Autodesk Inventor part; units mm, degrees
(part 3 of 6)
  arc A1155 (-87.7296, 1.38) -> (-88.2287, 1.0682) centre (-87.7298, 0.825) ccw
  arc A1156 (-88.2287, 1.0682) -> (-88.3213, 0.7604) centre (-87.3298, 0.63) ccw
  arc A1157 (-88.47, 0.63) -> (-88.3213, 0.7604) centre (-88.47, 0.78) ccw
  line L149 (-88.47, 0.63) -> (-88.9893, 0.63)
  arc A1158 (-89.138, 0.7604) -> (-88.9893, 0.63) centre (-88.9893, 0.78) ccw
  arc A1159 (-89.138, 0.7604) -> (-89.2306, 1.0682) centre (-90.1294, 0.63) ccw
  arc A1160 (-89.2306, 1.0682) -> (-89.7296, 1.38) centre (-89.7294, 0.825) ccw
  arc A1161 (-89.7296, 1.38) -> (-90.2287, 1.0682) centre (-89.7298, 0.825) ccw
  arc A1162 (-90.2287, 1.0682) -> (-90.3213, 0.7604) centre (-89.3298, 0.63) ccw
  arc A1163 (-90.47, 0.63) -> (-90.3213, 0.7604) centre (-90.47, 0.78) ccw
  line L150 (-90.47, 0.63) -> (-90.9893, 0.63)
  arc A1164 (-91.138, 0.7604) -> (-90.9893, 0.63) centre (-90.9893, 0.78) ccw
  arc A1165 (-91.138, 0.7604) -> (-91.2306, 1.0682) centre (-92.1294, 0.63) ccw
  arc A1166 (-91.2306, 1.0682) -> (-91.7296, 1.38) centre (-91.7294, 0.825) ccw
  arc A1167 (-91.7296, 1.38) -> (-92.2287, 1.0682) centre (-91.7298, 0.825) ccw
  arc A1168 (-92.2287, 1.0682) -> (-92.3213, 0.7604) centre (-91.3298, 0.63) ccw
  arc A1169 (-92.47, 0.63) -> (-92.3213, 0.7604) centre (-92.47, 0.78) ccw
  line L151 (-92.47, 0.63) -> (-92.9893, 0.63)
  arc A1170 (-93.138, 0.7604) -> (-92.9893, 0.63) centre (-92.9893, 0.78) ccw
  arc A1171 (-93.138, 0.7604) -> (-93.2306, 1.0682) centre (-94.1294, 0.63) ccw
  arc A1172 (-93.2306, 1.0682) -> (-93.7296, 1.38) centre (-93.7294, 0.825) ccw
  arc A1173 (-93.7296, 1.38) -> (-94.2287, 1.0682) centre (-93.7298, 0.825) ccw
  arc A1174 (-94.2287, 1.0682) -> (-94.3213, 0.7604) centre (-93.3298, 0.63) ccw
  arc A1175 (-94.47, 0.63) -> (-94.3213, 0.7604) centre (-94.47, 0.78) ccw
  line L152 (-94.47, 0.63) -> (-94.9893, 0.63)
  arc A1176 (-95.138, 0.7604) -> (-94.9893, 0.63) centre (-94.9893, 0.78) ccw
  arc A1177 (-95.138, 0.7604) -> (-95.2306, 1.0682) centre (-96.1294, 0.63) ccw
  arc A1178 (-95.2306, 1.0682) -> (-95.7296, 1.38) centre (-95.7294, 0.825) ccw
  arc A1179 (-95.7296, 1.38) -> (-96.2287, 1.0682) centre (-95.7298, 0.825) ccw
  arc A1180 (-96.2287, 1.0682) -> (-96.3213, 0.7604) centre (-95.3298, 0.63) ccw
  arc A1181 (-96.47, 0.63) -> (-96.3213, 0.7604) centre (-96.47, 0.78) ccw
  line L153 (-96.47, 0.63) -> (-96.9893, 0.63)
  arc A1182 (-97.138, 0.7604) -> (-96.9893, 0.63) centre (-96.9893, 0.78) ccw
  arc A1183 (-97.138, 0.7604) -> (-97.2306, 1.0682) centre (-98.1294, 0.63) ccw
  arc A1184 (-97.2306, 1.0682) -> (-97.7296, 1.38) centre (-97.7294, 0.825) ccw
  arc A1185 (-97.7296, 1.38) -> (-98.2287, 1.0682) centre (-97.7298, 0.825) ccw
  arc A1186 (-98.2287, 1.0682) -> (-98.3213, 0.7604) centre (-97.3298, 0.63) ccw
  arc A1187 (-98.47, 0.63) -> (-98.3213, 0.7604) centre (-98.47, 0.78) ccw
  line L154 (-98.47, 0.63) -> (-98.9893, 0.63)
  arc A1188 (-99.138, 0.7604) -> (-98.9893, 0.63) centre (-98.9893, 0.78) ccw
  arc A1189 (-99.138, 0.7604) -> (-99.2306, 1.0682) centre (-100.1294, 0.63) ccw
  arc A1190 (-99.2306, 1.0682) -> (-99.7296, 1.38) centre (-99.7294, 0.825) ccw
  arc A1191 (-99.7296, 1.38) -> (-100.2287, 1.0682) centre (-99.7298, 0.825) ccw
  arc A1192 (-100.2287, 1.0682) -> (-100.3213, 0.7604) centre (-99.3298, 0.63) ccw
  arc A1193 (-100.47, 0.63) -> (-100.3213, 0.7604) centre (-100.47, 0.78) ccw
  line L155 (-100.47, 0.63) -> (-100.9893, 0.63)
  arc A1194 (-101.138, 0.7604) -> (-100.9893, 0.63) centre (-100.9893, 0.78) ccw
  arc A1195 (-101.138, 0.7604) -> (-101.2306, 1.0682) centre (-102.1294, 0.63) ccw
  arc A1196 (-101.2306, 1.0682) -> (-101.7296, 1.38) centre (-101.7294, 0.825) ccw
  arc A1197 (-101.7296, 1.38) -> (-102.2287, 1.0682) centre (-101.7298, 0.825) ccw
  arc A1198 (-102.2287, 1.0682) -> (-102.3213, 0.7604) centre (-101.3298, 0.63) ccw
  arc A1199 (-102.47, 0.63) -> (-102.3213, 0.7604) centre (-102.47, 0.78) ccw
  line L156 (-102.47, 0.63) -> (-102.9893, 0.63)
  arc A1200 (-103.138, 0.7604) -> (-102.9893, 0.63) centre (-102.9893, 0.78) ccw
  arc A1201 (-103.138, 0.7604) -> (-103.2306, 1.0682) centre (-104.1294, 0.63) ccw
  arc A1202 (-103.2306, 1.0682) -> (-103.7296, 1.38) centre (-103.7294, 0.825) ccw
  arc A1203 (-103.7296, 1.38) -> (-104.2287, 1.0682) centre (-103.7298, 0.825) ccw
  arc A1204 (-104.2287, 1.0682) -> (-104.3213, 0.7604) centre (-103.3298, 0.63) ccw
  arc A1205 (-104.47, 0.63) -> (-104.3213, 0.7604) centre (-104.47, 0.78) ccw
  line L157 (-104.47, 0.63) -> (-104.9893, 0.63)
  arc A1206 (-105.138, 0.7604) -> (-104.9893, 0.63) centre (-104.9893, 0.78) ccw
  arc A1207 (-105.138, 0.7604) -> (-105.2306, 1.0682) centre (-106.1294, 0.63) ccw
  arc A1208 (-105.2306, 1.0682) -> (-105.7296, 1.38) centre (-105.7294, 0.825) ccw
  arc A1209 (-105.7296, 1.38) -> (-106.2287, 1.0682) centre (-105.7298, 0.825) ccw
  arc A1210 (-106.2287, 1.0682) -> (-106.3213, 0.7604) centre (-105.3298, 0.63) ccw
  arc A1211 (-106.47, 0.63) -> (-106.3213, 0.7604) centre (-106.47, 0.78) ccw
  line L158 (-106.47, 0.63) -> (-106.9893, 0.63)
  arc A1212 (-107.138, 0.7604) -> (-106.9893, 0.63) centre (-106.9893, 0.78) ccw
  arc A1213 (-107.138, 0.7604) -> (-107.2306, 1.0682) centre (-108.1294, 0.63) ccw
  arc A1214 (-107.2306, 1.0682) -> (-107.7296, 1.38) centre (-107.7294, 0.825) ccw
  arc A1215 (-107.7296, 1.38) -> (-108.2287, 1.0682) centre (-107.7298, 0.825) ccw
  arc A1216 (-108.2287, 1.0682) -> (-108.3213, 0.7604) centre (-107.3298, 0.63) ccw
  arc A1217 (-108.47, 0.63) -> (-108.3213, 0.7604) centre (-108.47, 0.78) ccw
  line L159 (-108.47, 0.63) -> (-108.9893, 0.63)
  arc A1218 (-109.138, 0.7604) -> (-108.9893, 0.63) centre (-108.9893, 0.78) ccw
  arc A1219 (-109.138, 0.7604) -> (-109.2306, 1.0682) centre (-110.1294, 0.63) ccw
  arc A1220 (-109.2306, 1.0682) -> (-109.7296, 1.38) centre (-109.7294, 0.825) ccw
  arc A1221 (-109.7296, 1.38) -> (-110.2287, 1.0682) centre (-109.7298, 0.825) ccw
  arc A1222 (-110.2287, 1.0682) -> (-110.3213, 0.7604) centre (-109.3298, 0.63) ccw
  arc A1223 (-110.47, 0.63) -> (-110.3213, 0.7604) centre (-110.47, 0.78) ccw
  line L160 (-110.47, 0.63) -> (-110.9893, 0.63)
  arc A1224 (-111.138, 0.7604) -> (-110.9893, 0.63) centre (-110.9893, 0.78) ccw
  arc A1225 (-111.138, 0.7604) -> (-111.2306, 1.0682) centre (-112.1294, 0.63) ccw
  arc A1226 (-111.2306, 1.0682) -> (-111.7296, 1.38) centre (-111.7294, 0.825) ccw
  arc A1227 (-111.7296, 1.38) -> (-112.2287, 1.0682) centre (-111.7298, 0.825) ccw
  arc A1228 (-112.2287, 1.0682) -> (-112.3213, 0.7604) centre (-111.3298, 0.63) ccw
  arc A1229 (-112.47, 0.63) -> (-112.3213, 0.7604) centre (-112.47, 0.78) ccw
  line L161 (-112.47, 0.63) -> (-112.9893, 0.63)
  arc A1230 (-113.138, 0.7604) -> (-112.9893, 0.63) centre (-112.9893, 0.78) ccw
  arc A1231 (-113.138, 0.7604) -> (-113.2306, 1.0682) centre (-114.1294, 0.63) ccw
  arc A1232 (-113.2306, 1.0682) -> (-113.7296, 1.38) centre (-113.7294, 0.825) ccw
  arc A1233 (-113.7296, 1.38) -> (-114.2287, 1.0682) centre (-113.7298, 0.825) ccw
  arc A1234 (-114.2287, 1.0682) -> (-114.3213, 0.7604) centre (-113.3298, 0.63) ccw
  arc A1235 (-114.47, 0.63) -> (-114.3213, 0.7604) centre (-114.47, 0.78) ccw
  line L162 (-114.47, 0.63) -> (-114.9893, 0.63)
  arc A1236 (-115.138, 0.7604) -> (-114.9893, 0.63) centre (-114.9893, 0.78) ccw
  arc A1237 (-115.138, 0.7604) -> (-115.2306, 1.0682) centre (-116.1294, 0.63) ccw
  arc A1238 (-115.2306, 1.0682) -> (-115.7296, 1.38) centre (-115.7294, 0.825) ccw
  arc A1239 (-115.7296, 1.38) -> (-116.2287, 1.0682) centre (-115.7298, 0.825) ccw
  arc A1240 (-116.2287, 1.0682) -> (-116.3213, 0.7604) centre (-115.3298, 0.63) ccw
  arc A1241 (-116.47, 0.63) -> (-116.3213, 0.7604) centre (-116.47, 0.78) ccw
  line L163 (-116.47, 0.63) -> (-116.9893, 0.63)
  arc A1242 (-117.138, 0.7604) -> (-116.9893, 0.63) centre (-116.9893, 0.78) ccw
  arc A1243 (-117.138, 0.7604) -> (-117.2306, 1.0682) centre (-118.1294, 0.63) ccw
  arc A1244 (-117.2306, 1.0682) -> (-117.7296, 1.38) centre (-117.7294, 0.825) ccw
  arc A1245 (-117.7296, 1.38) -> (-118.2287, 1.0682) centre (-117.7298, 0.825) ccw
  arc A1246 (-118.2287, 1.0682) -> (-118.3213, 0.7604) centre (-117.3298, 0.63) ccw
  arc A1247 (-118.47, 0.63) -> (-118.3213, 0.7604) centre (-118.47, 0.78) ccw
  line L164 (-118.47, 0.63) -> (-118.9893, 0.63)
  arc A1248 (-119.138, 0.7604) -> (-118.9893, 0.63) centre (-118.9893, 0.78) ccw
  arc A1249 (-119.138, 0.7604) -> (-119.2306, 1.0682) centre (-120.1294, 0.63) ccw
  arc A1250 (-119.2306, 1.0682) -> (-119.7296, 1.38) centre (-119.7294, 0.825) ccw
  arc A1251 (-119.7296, 1.38) -> (-120.2287, 1.0682) centre (-119.7298, 0.825) ccw
  arc A1252 (-120.2287, 1.0682) -> (-120.3213, 0.7604) centre (-119.3298, 0.63) ccw
  arc A1253 (-120.47, 0.63) -> (-120.3213, 0.7604) centre (-120.47, 0.78) ccw
  line L165 (-120.47, 0.63) -> (-120.9893, 0.63)
  arc A1254 (-121.138, 0.7604) -> (-120.9893, 0.63) centre (-120.9893, 0.78) ccw
  arc A1255 (-121.138, 0.7604) -> (-121.2306, 1.0682) centre (-122.1294, 0.63) ccw
  arc A1256 (-121.2306, 1.0682) -> (-121.7296, 1.38) centre (-121.7294, 0.825) ccw
  arc A1257 (-121.7296, 1.38) -> (-122.2287, 1.0682) centre (-121.7298, 0.825) ccw
  arc A1258 (-122.2287, 1.0682) -> (-122.3213, 0.7604) centre (-121.3298, 0.63) ccw
  arc A1259 (-122.47, 0.63) -> (-122.3213, 0.7604) centre (-122.47, 0.78) ccw
  line L166 (-122.47, 0.63) -> (-122.9893, 0.63)
  arc A1260 (-123.138, 0.7604) -> (-122.9893, 0.63) centre (-122.9893, 0.78) ccw
  arc A1261 (-123.138, 0.7604) -> (-123.2306, 1.0682) centre (-124.1294, 0.63) ccw
  arc A1262 (-123.2306, 1.0682) -> (-123.7296, 1.38) centre (-123.7294, 0.825) ccw
  arc A1263 (-123.7296, 1.38) -> (-124.2287, 1.0682) centre (-123.7298, 0.825) ccw
  arc A1264 (-124.2287, 1.0682) -> (-124.3213, 0.7604) centre (-123.3298, 0.63) ccw
  arc A1265 (-124.47, 0.63) -> (-124.3213, 0.7604) centre (-124.47, 0.78) ccw
  line L167 (-124.47, 0.63) -> (-124.9893, 0.63)
  arc A1266 (-125.138, 0.7604) -> (-124.9893, 0.63) centre (-124.9893, 0.78) ccw
  arc A1267 (-125.138, 0.7604) -> (-125.2306, 1.0682) centre (-126.1294, 0.63) ccw
  arc A1268 (-125.2306, 1.0682) -> (-125.7296, 1.38) centre (-125.7294, 0.825) ccw
  arc A1269 (-125.7296, 1.38) -> (-126.2287, 1.0682) centre (-125.7298, 0.825) ccw
  arc A1270 (-126.2287, 1.0682) -> (-126.3213, 0.7604) centre (-125.3298, 0.63) ccw
  arc A1271 (-126.47, 0.63) -> (-126.3213, 0.7604) centre (-126.47, 0.78) ccw
  line L168 (-126.47, 0.63) -> (-126.9893, 0.63)
  arc A1272 (-127.138, 0.7604) -> (-126.9893, 0.63) centre (-126.9893, 0.78) ccw
  arc A1273 (-127.138, 0.7604) -> (-127.2306, 1.0682) centre (-128.1294, 0.63) ccw
  arc A1274 (-127.2306, 1.0682) -> (-127.7296, 1.38) centre (-127.7294, 0.825) ccw
  arc A1275 (-127.7296, 1.38) -> (-128.2287, 1.0682) centre (-127.7298, 0.825) ccw
  arc A1276 (-128.2287, 1.0682) -> (-128.3213, 0.7604) centre (-127.3298, 0.63) ccw
  arc A1277 (-128.47, 0.63) -> (-128.3213, 0.7604) centre (-128.47, 0.78) ccw
  line L169 (-128.47, 0.63) -> (-128.9893, 0.63)
  arc A1278 (-129.138, 0.7604) -> (-128.9893, 0.63) centre (-128.9893, 0.78) ccw
  arc A1279 (-129.138, 0.7604) -> (-129.2306, 1.0682) centre (-130.1294, 0.63) ccw
  arc A1280 (-129.2306, 1.0682) -> (-129.7296, 1.38) centre (-129.7294, 0.825) ccw
  arc A1281 (-129.7296, 1.38) -> (-130.2287, 1.0682) centre (-129.7298, 0.825) ccw
  arc A1282 (-130.2287, 1.0682) -> (-130.3213, 0.7604) centre (-129.3298, 0.63) ccw
  arc A1283 (-130.47, 0.63) -> (-130.3213, 0.7604) centre (-130.47, 0.78) ccw
  line L170 (-130.47, 0.63) -> (-130.9893, 0.63)
  arc A1284 (-131.138, 0.7604) -> (-130.9893, 0.63) centre (-130.9893, 0.78) ccw
  arc A1285 (-131.138, 0.7604) -> (-131.2306, 1.0682) centre (-132.1294, 0.63) ccw
  arc A1286 (-131.2306, 1.0682) -> (-131.7296, 1.38) centre (-131.7294, 0.825) ccw
  arc A1287 (-131.7296, 1.38) -> (-132.2287, 1.0682) centre (-131.7298, 0.825) ccw
  arc A1288 (-132.2287, 1.0682) -> (-132.3213, 0.7604) centre (-131.3298, 0.63) ccw
  arc A1289 (-132.47, 0.63) -> (-132.3213, 0.7604) centre (-132.47, 0.78) ccw
  line L171 (-132.47, 0.63) -> (-132.9893, 0.63)
  arc A1290 (-133.138, 0.7604) -> (-132.9893, 0.63) centre (-132.9893, 0.78) ccw
  arc A1291 (-133.138, 0.7604) -> (-133.2306, 1.0682) centre (-134.1294, 0.63) ccw
  arc A1292 (-133.2306, 1.0682) -> (-133.7296, 1.38) centre (-133.7294, 0.825) ccw
  arc A1293 (-133.7296, 1.38) -> (-134.2287, 1.0682) centre (-133.7298, 0.825) ccw
  arc A1294 (-134.2287, 1.0682) -> (-134.3213, 0.7604) centre (-133.3298, 0.63) ccw
  arc A1295 (-134.47, 0.63) -> (-134.3213, 0.7604) centre (-134.47, 0.78) ccw
  line L172 (-134.47, 0.63) -> (-134.9893, 0.63)
  arc A1296 (-135.138, 0.7604) -> (-134.9893, 0.63) centre (-134.9893, 0.78) ccw
  arc A1297 (-135.138, 0.7604) -> (-135.2306, 1.0682) centre (-136.1294, 0.63) ccw
  arc A1298 (-135.2306, 1.0682) -> (-135.7296, 1.38) centre (-135.7294, 0.825) ccw
  arc A1299 (-135.7296, 1.38) -> (-136.2287, 1.0682) centre (-135.7298, 0.825) ccw
  arc A1300 (-136.2287, 1.0682) -> (-136.3213, 0.7604) centre (-135.3298, 0.63) ccw
  arc A1301 (-136.47, 0.63) -> (-136.3213, 0.7604) centre (-136.47, 0.78) ccw
  line L173 (-136.47, 0.63) -> (-136.9893, 0.63)
  arc A1302 (-137.138, 0.7604) -> (-136.9893, 0.63) centre (-136.9893, 0.78) ccw
  arc A1303 (-137.138, 0.7604) -> (-137.2306, 1.0682) centre (-138.1294, 0.63) ccw
  arc A1304 (-137.2306, 1.0682) -> (-137.7296, 1.38) centre (-137.7294, 0.825) ccw
  arc A1305 (-137.7296, 1.38) -> (-138.2287, 1.0682) centre (-137.7298, 0.825) ccw
  arc A1306 (-138.2287, 1.0682) -> (-138.3213, 0.7604) centre (-137.3298, 0.63) ccw
  arc A1307 (-138.47, 0.63) -> (-138.3213, 0.7604) centre (-138.47, 0.78) ccw
  line L174 (-138.47, 0.63) -> (-138.9893, 0.63)
  arc A1308 (-139.138, 0.7604) -> (-138.9893, 0.63) centre (-138.9893, 0.78) ccw
  arc A1309 (-139.138, 0.7604) -> (-139.2306, 1.0682) centre (-140.1294, 0.63) ccw
  arc A1310 (-139.2306, 1.0682) -> (-139.7296, 1.38) centre (-139.7294, 0.825) ccw
  arc A1311 (-139.7296, 1.38) -> (-140.2287, 1.0682) centre (-139.7298, 0.825) ccw
  arc A1312 (-140.2287, 1.0682) -> (-140.3213, 0.7604) centre (-139.3298, 0.63) ccw
  arc A1313 (-140.47, 0.63) -> (-140.3213, 0.7604) centre (-140.47, 0.78) ccw
  line L175 (-140.47, 0.63) -> (-140.9893, 0.63)
  arc A1314 (-141.138, 0.7604) -> (-140.9893, 0.63) centre (-140.9893, 0.78) ccw
  arc A1315 (-141.138, 0.7604) -> (-141.2306, 1.0682) centre (-142.1294, 0.63) ccw
  arc A1316 (-141.2306, 1.0682) -> (-141.7296, 1.38) centre (-141.7294, 0.825) ccw
  arc A1317 (-141.7296, 1.38) -> (-142.2287, 1.0682) centre (-141.7298, 0.825) ccw
  arc A1318 (-142.2287, 1.0682) -> (-142.3213, 0.7604) centre (-141.3298, 0.63) ccw
  arc A1319 (-142.47, 0.63) -> (-142.3213, 0.7604) centre (-142.47, 0.78) ccw
  line L176 (-142.47, 0.63) -> (-142.9893, 0.63)
  arc A1320 (-143.138, 0.7604) -> (-142.9893, 0.63) centre (-142.9893, 0.78) ccw
  arc A1321 (-143.138, 0.7604) -> (-143.2306, 1.0682) centre (-144.1294, 0.63) ccw
  arc A1322 (-143.2306, 1.0682) -> (-143.7296, 1.38) centre (-143.7294, 0.825) ccw
  arc A1323 (-143.7296, 1.38) -> (-144.2287, 1.0682) centre (-143.7298, 0.825) ccw
  arc A1324 (-144.2287, 1.0682) -> (-144.3213, 0.7604) centre (-143.3298, 0.63) ccw
  arc A1325 (-144.47, 0.63) -> (-144.3213, 0.7604) centre (-144.47, 0.78) ccw
  line L177 (-144.47, 0.63) -> (-144.9893, 0.63)
  arc A1326 (-145.138, 0.7604) -> (-144.9893, 0.63) centre (-144.9893, 0.78) ccw
  arc A1327 (-145.138, 0.7604) -> (-145.2306, 1.0682) centre (-146.1294, 0.63) ccw
  arc A1328 (-145.2306, 1.0682) -> (-145.7296, 1.38) centre (-145.7294, 0.825) ccw
  arc A1329 (-145.7296, 1.38) -> (-146.2287, 1.0682) centre (-145.7298, 0.825) ccw
  arc A1330 (-146.2287, 1.0682) -> (-146.3213, 0.7604) centre (-145.3298, 0.63) ccw
  arc A1331 (-146.47, 0.63) -> (-146.3213, 0.7604) centre (-146.47, 0.78) ccw
  line L178 (-146.47, 0.63) -> (-146.9893, 0.63)
  arc A1332 (-147.138, 0.7604) -> (-146.9893, 0.63) centre (-146.9893, 0.78) ccw
  arc A1333 (-147.138, 0.7604) -> (-147.2306, 1.0682) centre (-148.1294, 0.63) ccw
  arc A1334 (-147.2306, 1.0682) -> (-147.7296, 1.38) centre (-147.7294, 0.825) ccw
  arc A1335 (-147.7296, 1.38) -> (-148.2287, 1.0682) centre (-147.7298, 0.825) ccw
  arc A1336 (-148.2287, 1.0682) -> (-148.3213, 0.7604) centre (-147.3298, 0.63) ccw
  arc A1337 (-148.47, 0.63) -> (-148.3213, 0.7604) centre (-148.47, 0.78) ccw
  line L179 (-148.47, 0.63) -> (-148.9893, 0.63)
  arc A1338 (-149.138, 0.7604) -> (-148.9893, 0.63) centre (-148.9893, 0.78) ccw
  arc A1339 (-149.138, 0.7604) -> (-149.2306, 1.0682) centre (-150.1294, 0.63) ccw
  arc A1340 (-149.2306, 1.0682) -> (-149.7296, 1.38) centre (-149.7294, 0.825) ccw
  arc A1341 (-149.7296, 1.38) -> (-150.2287, 1.0682) centre (-149.7298, 0.825) ccw
  arc A1342 (-150.2287, 1.0682) -> (-150.3213, 0.7604) centre (-149.3298, 0.63) ccw
  arc A1343 (-150.47, 0.63) -> (-150.3213, 0.7604) centre (-150.47, 0.78) ccw
  line L180 (-150.47, 0.63) -> (-150.9893, 0.63)
  arc A1344 (-151.138, 0.7604) -> (-150.9893, 0.63) centre (-150.9893, 0.78) ccw
  arc A1345 (-151.138, 0.7604) -> (-151.2306, 1.0682) centre (-152.1294, 0.63) ccw
  arc A1346 (-151.2306, 1.0682) -> (-151.7296, 1.38) centre (-151.7294, 0.825) ccw
  arc A1347 (-151.7296, 1.38) -> (-152.2287, 1.0682) centre (-151.7298, 0.825) ccw
  arc A1348 (-152.2287, 1.0682) -> (-152.3213, 0.7604) centre (-151.3298, 0.63) ccw
  arc A1349 (-152.47, 0.63) -> (-152.3213, 0.7604) centre (-152.47, 0.78) ccw
  line L181 (-152.47, 0.63) -> (-152.9893, 0.63)
  arc A1350 (-153.138, 0.7604) -> (-152.9893, 0.63) centre (-152.9893, 0.78) ccw
  arc A1351 (-153.138, 0.7604) -> (-153.2306, 1.0682) centre (-154.1294, 0.63) ccw
  arc A1352 (-153.2306, 1.0682) -> (-153.7296, 1.38) centre (-153.7294, 0.825) ccw
  arc A1353 (-153.7296, 1.38) -> (-154.2287, 1.0682) centre (-153.7298, 0.825) ccw
  arc A1354 (-154.2287, 1.0682) -> (-154.3213, 0.7604) centre (-153.3298, 0.63) ccw
  arc A1355 (-154.47, 0.63) -> (-154.3213, 0.7604) centre (-154.47, 0.78) ccw
  line L182 (-154.47, 0.63) -> (-154.9893, 0.63)
  arc A1356 (-155.138, 0.7604) -> (-154.9893, 0.63) centre (-154.9893, 0.78) ccw
  arc A1357 (-155.138, 0.7604) -> (-155.2306, 1.0682) centre (-156.1294, 0.63) ccw
  arc A1358 (-155.2306, 1.0682) -> (-155.7296, 1.38) centre (-155.7294, 0.825) ccw
  arc A1359 (-155.7296, 1.38) -> (-156.2287, 1.0682) centre (-155.7298, 0.825) ccw
  arc A1360 (-156.2287, 1.0682) -> (-156.3213, 0.7604) centre (-155.3298, 0.63) ccw
  arc A1361 (-156.47, 0.63) -> (-156.3213, 0.7604) centre (-156.47, 0.78) ccw
  line L183 (-156.47, 0.63) -> (-156.9893, 0.63)
  arc A1362 (-157.138, 0.7604) -> (-156.9893, 0.63) centre (-156.9893, 0.78) ccw
  arc A1363 (-157.138, 0.7604) -> (-157.2306, 1.0682) centre (-158.1294, 0.63) ccw
  arc A1364 (-157.2306, 1.0682) -> (-157.7296, 1.38) centre (-157.7294, 0.825) ccw
  arc A1365 (-157.7296, 1.38) -> (-158.2287, 1.0682) centre (-157.7298, 0.825) ccw
  arc A1366 (-158.2287, 1.0682) -> (-158.3213, 0.7604) centre (-157.3298, 0.63) ccw
  arc A1367 (-158.47, 0.63) -> (-158.3213, 0.7604) centre (-158.47, 0.78) ccw
  line L184 (-158.47, 0.63) -> (-158.9893, 0.63)
  arc A1368 (-159.138, 0.7604) -> (-158.9893, 0.63) centre (-158.9893, 0.78) ccw
  arc A1369 (-159.138, 0.7604) -> (-159.2306, 1.0682) centre (-160.1294, 0.63) ccw
  arc A1370 (-159.2306, 1.0682) -> (-159.7296, 1.38) centre (-159.7294, 0.825) ccw
  arc A1371 (-159.7296, 1.38) -> (-160.2287, 1.0682) centre (-159.7298, 0.825) ccw
  arc A1372 (-160.2287, 1.0682) -> (-160.3213, 0.7604) centre (-159.3298, 0.63) ccw
  arc A1373 (-160.47, 0.63) -> (-160.3213, 0.7604) centre (-160.47, 0.78) ccw
  line L185 (-160.47, 0.63) -> (-160.9893, 0.63)
  arc A1374 (-161.138, 0.7604) -> (-160.9893, 0.63) centre (-160.9893, 0.78) ccw
  arc A1375 (-161.138, 0.7604) -> (-161.2306, 1.0682) centre (-162.1294, 0.63) ccw
  arc A1376 (-161.2306, 1.0682) -> (-161.7296, 1.38) centre (-161.7294, 0.825) ccw
  arc A1377 (-161.7296, 1.38) -> (-162.2287, 1.0682) centre (-161.7298, 0.825) ccw
  arc A1378 (-162.2287, 1.0682) -> (-162.3213, 0.7604) centre (-161.3298, 0.63) ccw
  arc A1379 (-162.47, 0.63) -> (-162.3213, 0.7604) centre (-162.47, 0.78) ccw
  line L186 (-162.47, 0.63) -> (-162.9893, 0.63)
  arc A1380 (-163.138, 0.7604) -> (-162.9893, 0.63) centre (-162.9893, 0.78) ccw
  arc A1381 (-163.138, 0.7604) -> (-163.2306, 1.0682) centre (-164.1294, 0.63) ccw
  arc A1382 (-163.2306, 1.0682) -> (-163.7296, 1.38) centre (-163.7294, 0.825) ccw
  arc A1383 (-163.7296, 1.38) -> (-164.2287, 1.0682) centre (-163.7298, 0.825) ccw
  arc A1384 (-164.2287, 1.0682) -> (-164.3213, 0.7604) centre (-163.3298, 0.63) ccw
  arc A1385 (-164.47, 0.63) -> (-164.3213, 0.7604) centre (-164.47, 0.78) ccw
  line L187 (-164.47, 0.63) -> (-164.9893, 0.63)
  arc A1386 (-165.138, 0.7604) -> (-164.9893, 0.63) centre (-164.9893, 0.78) ccw
  arc A1387 (-165.138, 0.7604) -> (-165.2306, 1.0682) centre (-166.1294, 0.63) ccw
  arc A1388 (-165.2306, 1.0682) -> (-165.7296, 1.38) centre (-165.7294, 0.825) ccw
  arc A1389 (-165.7296, 1.38) -> (-166.2287, 1.0682) centre (-165.7298, 0.825) ccw
  arc A1390 (-166.2287, 1.0682) -> (-166.3213, 0.7604) centre (-165.3298, 0.63) ccw
  arc A1391 (-166.47, 0.63) -> (-166.3213, 0.7604) centre (-166.47, 0.78) ccw
  line L188 (-166.47, 0.63) -> (-166.9893, 0.63)
  arc A1392 (-167.138, 0.7604) -> (-166.9893, 0.63) centre (-166.9893, 0.78) ccw
  arc A1393 (-167.138, 0.7604) -> (-167.2306, 1.0682) centre (-168.1294, 0.63) ccw
  arc A1394 (-167.2306, 1.0682) -> (-167.7296, 1.38) centre (-167.7294, 0.825) ccw
  arc A1395 (-167.7296, 1.38) -> (-168.2287, 1.0682) centre (-167.7298, 0.825) ccw
  arc A1396 (-168.2287, 1.0682) -> (-168.3213, 0.7604) centre (-167.3298, 0.63) ccw
  arc A1397 (-168.47, 0.63) -> (-168.3213, 0.7604) centre (-168.47, 0.78) ccw
  line L189 (-168.47, 0.63) -> (-168.9893, 0.63)
  arc A1398 (-169.138, 0.7604) -> (-168.9893, 0.63) centre (-168.9893, 0.78) ccw
  arc A1399 (-169.138, 0.7604) -> (-169.2306, 1.0682) centre (-170.1294, 0.63) ccw
  arc A1400 (-169.2306, 1.0682) -> (-169.7296, 1.38) centre (-169.7294, 0.825) ccw
  arc A1401 (-169.7296, 1.38) -> (-170.2287, 1.0682) centre (-169.7298, 0.825) ccw
  arc A1402 (-170.2287, 1.0682) -> (-170.3213, 0.7604) centre (-169.3298, 0.63) ccw
  arc A1403 (-170.47, 0.63) -> (-170.3213, 0.7604) centre (-170.47, 0.78) ccw
  line L190 (-170.47, 0.63) -> (-170.9893, 0.63)
  arc A1404 (-171.138, 0.7604) -> (-170.9893, 0.63) centre (-170.9893, 0.78) ccw
  arc A1405 (-171.138, 0.7604) -> (-171.2306, 1.0682) centre (-172.1294, 0.63) ccw
  arc A1406 (-171.2306, 1.0682) -> (-171.7296, 1.38) centre (-171.7294, 0.825) ccw
  arc A1407 (-171.7296, 1.38) -> (-172.2287, 1.0682) centre (-171.7298, 0.825) ccw
  arc A1408 (-172.2287, 1.0682) -> (-172.3213, 0.7604) centre (-171.3298, 0.63) ccw
  arc A1409 (-172.47, 0.63) -> (-172.3213, 0.7604) centre (-172.47, 0.78) ccw
  line L191 (-172.47, 0.63) -> (-172.9893, 0.63)
  arc A1410 (-173.138, 0.7604) -> (-172.9893, 0.63) centre (-172.9893, 0.78) ccw
  arc A1411 (-173.138, 0.7604) -> (-173.2306, 1.0682) centre (-174.1294, 0.63) ccw
  arc A1412 (-173.2306, 1.0682) -> (-173.7296, 1.38) centre (-173.7294, 0.825) ccw
  arc A1413 (-173.7296, 1.38) -> (-174.2287, 1.0682) centre (-173.7298, 0.825) ccw
  arc A1414 (-174.2287, 1.0682) -> (-174.3213, 0.7604) centre (-173.3298, 0.63) ccw
  arc A1415 (-174.47, 0.63) -> (-174.3213, 0.7604) centre (-174.47, 0.78) ccw
  line L192 (-174.47, 0.63) -> (-174.9893, 0.63)
  arc A1416 (-175.138, 0.7604) -> (-174.9893, 0.63) centre (-174.9893, 0.78) ccw
  arc A1417 (-175.138, 0.7604) -> (-175.2306, 1.0682) centre (-176.1294, 0.63) ccw
  arc A1418 (-175.2306, 1.0682) -> (-175.7296, 1.38) centre (-175.7294, 0.825) ccw
  arc A1419 (-175.7296, 1.38) -> (-176.2287, 1.0682) centre (-175.7298, 0.825) ccw
  arc A1420 (-176.2287, 1.0682) -> (-176.3213, 0.7604) centre (-175.3298, 0.63) ccw
  arc A1421 (-176.47, 0.63) -> (-176.3213, 0.7604) centre (-176.47, 0.78) ccw
  line L193 (-176.47, 0.63) -> (-176.9893, 0.63)
  arc A1422 (-177.138, 0.7604) -> (-176.9893, 0.63) centre (-176.9893, 0.78) ccw
  arc A1423 (-177.138, 0.7604) -> (-177.2306, 1.0682) centre (-178.1294, 0.63) ccw
  arc A1424 (-177.2306, 1.0682) -> (-177.7296, 1.38) centre (-177.7294, 0.825) ccw
  arc A1425 (-177.7296, 1.38) -> (-178.2287, 1.0682) centre (-177.7298, 0.825) ccw
  arc A1426 (-178.2287, 1.0682) -> (-178.3213, 0.7604) centre (-177.3298, 0.63) ccw
  arc A1427 (-178.47, 0.63) -> (-178.3213, 0.7604) centre (-178.47, 0.78) ccw
  line L194 (-178.47, 0.63) -> (-178.9893, 0.63)
  arc A1428 (-179.138, 0.7604) -> (-178.9893, 0.63) centre (-178.9893, 0.78) ccw
  arc A1429 (-179.138, 0.7604) -> (-179.2306, 1.0682) centre (-180.1294, 0.63) ccw
  arc A1430 (-179.2306, 1.0682) -> (-179.7296, 1.38) centre (-179.7294, 0.825) ccw
  arc A1431 (-179.7296, 1.38) -> (-180.2287, 1.0682) centre (-179.7298, 0.825) ccw
  arc A1432 (-180.2287, 1.0682) -> (-180.3213, 0.7604) centre (-179.3298, 0.63) ccw
  arc A1433 (-180.47, 0.63) -> (-180.3213, 0.7604) centre (-180.47, 0.78) ccw
  line L195 (-180.47, 0.63) -> (-180.9893, 0.63)
  arc A1434 (-181.138, 0.7604) -> (-180.9893, 0.63) centre (-180.9893, 0.78) ccw
  arc A1435 (-181.138, 0.7604) -> (-181.2306, 1.0682) centre (-182.1294, 0.63) ccw
  arc A1436 (-181.2306, 1.0682) -> (-181.7296, 1.38) centre (-181.7294, 0.825) ccw
  arc A1437 (-181.7296, 1.38) -> (-182.2287, 1.0682) centre (-181.7298, 0.825) ccw
  arc A1438 (-182.2287, 1.0682) -> (-182.3213, 0.7604) centre (-181.3298, 0.63) ccw
  arc A1439 (-182.47, 0.63) -> (-182.3213, 0.7604) centre (-182.47, 0.78) ccw
  line L196 (-182.47, 0.63) -> (-182.9893, 0.63)
  arc A1440 (-183.138, 0.7604) -> (-182.9893, 0.63) centre (-182.9893, 0.78) ccw
  arc A1441 (-183.138, 0.7604) -> (-183.2306, 1.0682) centre (-184.1294, 0.63) ccw
  arc A1442 (-183.2306, 1.0682) -> (-183.7296, 1.38) centre (-183.7294, 0.825) ccw
  arc A1443 (-183.7296, 1.38) -> (-184.2287, 1.0682) centre (-183.7298, 0.825) ccw
  arc A1444 (-184.2287, 1.0682) -> (-184.3213, 0.7604) centre (-183.3298, 0.63) ccw
  arc A1445 (-184.47, 0.63) -> (-184.3213, 0.7604) centre (-184.47, 0.78) ccw
  line L197 (-184.47, 0.63) -> (-184.9893, 0.63)
  arc A1446 (-185.138, 0.7604) -> (-184.9893, 0.63) centre (-184.9893, 0.78) ccw
  arc A1447 (-185.138, 0.7604) -> (-185.2306, 1.0682) centre (-186.1294, 0.63) ccw
  arc A1448 (-185.2306, 1.0682) -> (-185.7296, 1.38) centre (-185.7294, 0.825) ccw
  arc A1449 (-185.7296, 1.38) -> (-186.2287, 1.0682) centre (-185.7298, 0.825) ccw
  arc A1450 (-186.2287, 1.0682) -> (-186.3213, 0.7604) centre (-185.3298, 0.63) ccw
  arc A1451 (-186.47, 0.63) -> (-186.3213, 0.7604) centre (-186.47, 0.78) ccw
  line L198 (-186.47, 0.63) -> (-186.9893, 0.63)
  arc A1452 (-187.138, 0.7604) -> (-186.9893, 0.63) centre (-186.9893, 0.78) ccw
  arc A1453 (-187.138, 0.7604) -> (-187.2306, 1.0682) centre (-188.1294, 0.63) ccw
  arc A1454 (-187.2306, 1.0682) -> (-187.7296, 1.38) centre (-187.7294, 0.825) ccw
  arc A1455 (-187.7296, 1.38) -> (-188.2287, 1.0682) centre (-187.7298, 0.825) ccw
  arc A1456 (-188.2287, 1.0682) -> (-188.3213, 0.7604) centre (-187.3298, 0.63) ccw
  arc A1457 (-188.47, 0.63) -> (-188.3213, 0.7604) centre (-188.47, 0.78) ccw
  line L199 (-188.47, 0.63) -> (-188.9893, 0.63)
  arc A1458 (-189.138, 0.7604) -> (-188.9893, 0.63) centre (-188.9893, 0.78) ccw
  arc A1459 (-189.138, 0.7604) -> (-189.2306, 1.0682) centre (-190.1294, 0.63) ccw
  arc A1460 (-189.2306, 1.0682) -> (-189.7296, 1.38) centre (-189.7294, 0.825) ccw
  arc A1461 (-189.7296, 1.38) -> (-190.2287, 1.0682) centre (-189.7298, 0.825) ccw
  arc A1462 (-190.2287, 1.0682) -> (-190.3213, 0.7604) centre (-189.3298, 0.63) ccw
  arc A1463 (-190.47, 0.63) -> (-190.3213, 0.7604) centre (-190.47, 0.78) ccw
  line L200 (-190.47, 0.63) -> (-190.9893, 0.63)
  arc A1464 (-191.138, 0.7604) -> (-190.9893, 0.63) centre (-190.9893, 0.78) ccw
  arc A1465 (-191.138, 0.7604) -> (-191.2306, 1.0682) centre (-192.1294, 0.63) ccw
  arc A1466 (-191.2306, 1.0682) -> (-191.7296, 1.38) centre (-191.7294, 0.825) ccw
  arc A1467 (-191.7296, 1.38) -> (-192.2287, 1.0682) centre (-191.7298, 0.825) ccw
  arc A1468 (-192.2287, 1.0682) -> (-192.3213, 0.7604) centre (-191.3298, 0.63) ccw
  arc A1469 (-192.47, 0.63) -> (-192.3213, 0.7604) centre (-192.47, 0.78) ccw
  line L201 (-192.47, 0.63) -> (-192.9893, 0.63)
  arc A1470 (-193.138, 0.7604) -> (-192.9893, 0.63) centre (-192.9893, 0.78) ccw
  arc A1471 (-193.138, 0.7604) -> (-193.2306, 1.0682) centre (-194.1294, 0.63) ccw
  arc A1472 (-193.2306, 1.0682) -> (-193.7296, 1.38) centre (-193.7294, 0.825) ccw
  arc A1473 (-193.7296, 1.38) -> (-194.2287, 1.0682) centre (-193.7298, 0.825) ccw
  arc A1474 (-194.2287, 1.0682) -> (-194.3213, 0.7604) centre (-193.3298, 0.63) ccw
  arc A1475 (-194.47, 0.63) -> (-194.3213, 0.7604) centre (-194.47, 0.78) ccw
  line L202 (-194.47, 0.63) -> (-194.9893, 0.63)
  arc A1476 (-195.138, 0.7604) -> (-194.9893, 0.63) centre (-194.9893, 0.78) ccw
  arc A1477 (-195.138, 0.7604) -> (-195.2306, 1.0682) centre (-196.1294, 0.63) ccw
  arc A1478 (-195.2306, 1.0682) -> (-195.7296, 1.38) centre (-195.7294, 0.825) ccw
  arc A1479 (-195.7296, 1.38) -> (-196.2287, 1.0682) centre (-195.7298, 0.825) ccw
  arc A1480 (-196.2287, 1.0682) -> (-196.3213, 0.7604) centre (-195.3298, 0.63) ccw
  arc A1481 (-196.47, 0.63) -> (-196.3213, 0.7604) centre (-196.47, 0.78) ccw
  line L203 (-196.47, 0.63) -> (-196.9893, 0.63)
  arc A1482 (-197.138, 0.7604) -> (-196.9893, 0.63) centre (-196.9893, 0.78) ccw
  arc A1483 (-197.138, 0.7604) -> (-197.2306, 1.0682) centre (-198.1294, 0.63) ccw
  arc A1484 (-197.2306, 1.0682) -> (-197.7296, 1.38) centre (-197.7294, 0.825) ccw
  arc A1485 (-197.7296, 1.38) -> (-198.2287, 1.0682) centre (-197.7298, 0.825) ccw
  arc A1486 (-198.2287, 1.0682) -> (-198.3213, 0.7604) centre (-197.3298, 0.63) ccw
  arc A1487 (-198.47, 0.63) -> (-198.3213, 0.7604) centre (-198.47, 0.78) ccw
  line L204 (-198.47, 0.63) -> (-198.9893, 0.63)
  arc A1488 (-199.138, 0.7604) -> (-198.9893, 0.63) centre (-198.9893, 0.78) ccw
  arc A1489 (-199.138, 0.7604) -> (-199.2306, 1.0682) centre (-200.1294, 0.63) ccw
  arc A1490 (-199.2306, 1.0682) -> (-199.7296, 1.38) centre (-199.7294, 0.825) ccw
  arc A1491 (-199.7296, 1.38) -> (-200.2287, 1.0682) centre (-199.7298, 0.825) ccw
  arc A1492 (-200.2287, 1.0682) -> (-200.3213, 0.7604) centre (-199.3298, 0.63) ccw
  arc A1493 (-200.47, 0.63) -> (-200.3213, 0.7604) centre (-200.47, 0.78) ccw
  line L205 (-200.47, 0.63) -> (-200.9893, 0.63)
  arc A1494 (-201.138, 0.7604) -> (-200.9893, 0.63) centre (-200.9893, 0.78) ccw
  arc A1495 (-201.138, 0.7604) -> (-201.2306, 1.0682) centre (-202.1294, 0.63) ccw
  arc A1496 (-201.2306, 1.0682) -> (-201.7296, 1.38) centre (-201.7294, 0.825) ccw
  arc A1497 (-201.7296, 1.38) -> (-202.2287, 1.0682) centre (-201.7298, 0.825) ccw
  arc A1498 (-202.2287, 1.0682) -> (-202.3213, 0.7604) centre (-201.3298, 0.63) ccw
  arc A1499 (-202.47, 0.63) -> (-202.3213, 0.7604) centre (-202.47, 0.78) ccw
  line L206 (-202.47, 0.63) -> (-202.9893, 0.63)
  arc A1500 (-203.138, 0.7604) -> (-202.9893, 0.63) centre (-202.9893, 0.78) ccw
  arc A1501 (-203.138, 0.7604) -> (-203.2306, 1.0682) centre (-204.1294, 0.63) ccw
  arc A1502 (-203.2306, 1.0682) -> (-203.7296, 1.38) centre (-203.7294, 0.825) ccw
  arc A1503 (-203.7296, 1.38) -> (-204.2287, 1.0682) centre (-203.7298, 0.825) ccw
  arc A1504 (-204.2287, 1.0682) -> (-204.3213, 0.7604) centre (-203.3298, 0.63) ccw
  arc A1505 (-204.47, 0.63) -> (-204.3213, 0.7604) centre (-204.47, 0.78) ccw
  line L207 (-204.47, 0.63) -> (-204.9893, 0.63)
  arc A1506 (-205.138, 0.7604) -> (-204.9893, 0.63) centre (-204.9893, 0.78) ccw
  arc A1507 (-205.138, 0.7604) -> (-205.2306, 1.0682) centre (-206.1294, 0.63) ccw
  arc A1508 (-205.2306, 1.0682) -> (-205.7296, 1.38) centre (-205.7294, 0.825) ccw
  arc A1509 (-205.7296, 1.38) -> (-206.2287, 1.0682) centre (-205.7298, 0.825) ccw
  arc A1510 (-206.2287, 1.0682) -> (-206.3213, 0.7604) centre (-205.3298, 0.63) ccw
  arc A1511 (-206.47, 0.63) -> (-206.3213, 0.7604) centre (-206.47, 0.78) ccw
  line L208 (-206.47, 0.63) -> (-206.9893, 0.63)
  arc A1512 (-207.138, 0.7604) -> (-206.9893, 0.63) centre (-206.9893, 0.78) ccw
  arc A1513 (-207.138, 0.7604) -> (-207.2306, 1.0682) centre (-208.1294, 0.63) ccw
  arc A1514 (-207.2306, 1.0682) -> (-207.7296, 1.38) centre (-207.7294, 0.825) ccw
  arc A1515 (-207.7296, 1.38) -> (-208.2287, 1.0682) centre (-207.7298, 0.825) ccw
  arc A1516 (-208.2287, 1.0682) -> (-208.3213, 0.7604) centre (-207.3298, 0.63) ccw
  arc A1517 (-208.47, 0.63) -> (-208.3213, 0.7604) centre (-208.47, 0.78) ccw
  line L209 (-208.47, 0.63) -> (-208.9893, 0.63)
  arc A1518 (-209.138, 0.7604) -> (-208.9893, 0.63) centre (-208.9893, 0.78) ccw
  arc A1519 (-209.138, 0.7604) -> (-209.2306, 1.0682) centre (-210.1294, 0.63) ccw
  arc A1520 (-209.2306, 1.0682) -> (-209.7296, 1.38) centre (-209.7294, 0.825) ccw
  arc A1521 (-209.7296, 1.38) -> (-210.2287, 1.0682) centre (-209.7298, 0.825) ccw
  arc A1522 (-210.2287, 1.0682) -> (-210.3213, 0.7604) centre (-209.3298, 0.63) ccw
  arc A1523 (-210.47, 0.63) -> (-210.3213, 0.7604) centre (-210.47, 0.78) ccw
  line L210 (-210.47, 0.63) -> (-210.9893, 0.63)
  arc A1524 (-211.138, 0.7604) -> (-210.9893, 0.63) centre (-210.9893, 0.78) ccw
  arc A1525 (-211.138, 0.7604) -> (-211.2306, 1.0682) centre (-212.1294, 0.63) ccw
  arc A1526 (-211.2306, 1.0682) -> (-211.7296, 1.38) centre (-211.7294, 0.825) ccw
  arc A1527 (-211.7296, 1.38) -> (-212.2287, 1.0682) centre (-211.7298, 0.825) ccw
  arc A1528 (-212.2287, 1.0682) -> (-212.3213, 0.7604) centre (-211.3298, 0.63) ccw
  arc A1529 (-212.47, 0.63) -> (-212.3213, 0.7604) centre (-212.47, 0.78) ccw
  line L211 (-212.47, 0.63) -> (-212.9893, 0.63)
  arc A1530 (-213.138, 0.7604) -> (-212.9893, 0.63) centre (-212.9893, 0.78) ccw
  arc A1531 (-213.138, 0.7604) -> (-213.2306, 1.0682) centre (-214.1294, 0.63) ccw
  arc A1532 (-213.2306, 1.0682) -> (-213.7296, 1.38) centre (-213.7294, 0.825) ccw
  arc A1533 (-213.7296, 1.38) -> (-214.2287, 1.0682) centre (-213.7298, 0.825) ccw
  arc A1534 (-214.2287, 1.0682) -> (-214.3213, 0.7604) centre (-213.3298, 0.63) ccw
  arc A1535 (-214.47, 0.63) -> (-214.3213, 0.7604) centre (-214.47, 0.78) ccw
  line L212 (-214.47, 0.63) -> (-214.9893, 0.63)
  arc A1536 (-215.138, 0.7604) -> (-214.9893, 0.63) centre (-214.9893, 0.78) ccw
  arc A1537 (-215.138, 0.7604) -> (-215.2306, 1.0682) centre (-216.1294, 0.63) ccw
  arc A1538 (-215.2306, 1.0682) -> (-215.7296, 1.38) centre (-215.7294, 0.825) ccw
  arc A1539 (-215.7296, 1.38) -> (-216.2287, 1.0682) centre (-215.7298, 0.825) ccw
  arc A1540 (-216.2287, 1.0682) -> (-216.3213, 0.7604) centre (-215.3298, 0.63) ccw
  arc A1541 (-216.47, 0.63) -> (-216.3213, 0.7604) centre (-216.47, 0.78) ccw
  line L213 (-216.47, 0.63) -> (-216.9893, 0.63)
  arc A1542 (-217.138, 0.7604) -> (-216.9893, 0.63) centre (-216.9893, 0.78) ccw
  arc A1543 (-217.138, 0.7604) -> (-217.2306, 1.0682) centre (-218.1294, 0.63) ccw
  arc A1544 (-217.2306, 1.0682) -> (-217.7296, 1.38) centre (-217.7294, 0.825) ccw
  arc A1545 (-217.7296, 1.38) -> (-218.2287, 1.0682) centre (-217.7298, 0.825) ccw
  arc A1546 (-218.2287, 1.0682) -> (-218.3213, 0.7604) centre (-217.3298, 0.63) ccw
  arc A1547 (-218.47, 0.63) -> (-218.3213, 0.7604) centre (-218.47, 0.78) ccw
  line L214 (-218.47, 0.63) -> (-218.9893, 0.63)
  arc A1548 (-219.138, 0.7604) -> (-218.9893, 0.63) centre (-218.9893, 0.78) ccw
  arc A1549 (-219.138, 0.7604) -> (-219.2306, 1.0682) centre (-220.1294, 0.63) ccw
  arc A1550 (-219.2306, 1.0682) -> (-219.7296, 1.38) centre (-219.7294, 0.825) ccw
  arc A1551 (-219.7296, 1.38) -> (-220.2287, 1.0682) centre (-219.7298, 0.825) ccw
  arc A1552 (-220.2287, 1.0682) -> (-220.3213, 0.7604) centre (-219.3298, 0.63) ccw
  arc A1553 (-220.47, 0.63) -> (-220.3213, 0.7604) centre (-220.47, 0.78) ccw
  line L215 (-220.47, 0.63) -> (-220.9893, 0.63)
  arc A1554 (-221.138, 0.7604) -> (-220.9893, 0.63) centre (-220.9893, 0.78) ccw
  arc A1555 (-221.138, 0.7604) -> (-221.2306, 1.0682) centre (-222.1294, 0.63) ccw
  arc A1556 (-221.2306, 1.0682) -> (-221.7296, 1.38) centre (-221.7294, 0.825) ccw
  arc A1557 (-221.7296, 1.38) -> (-222.2287, 1.0682) centre (-221.7298, 0.825) ccw
  arc A1558 (-222.2287, 1.0682) -> (-222.3213, 0.7604) centre (-221.3298, 0.63) ccw
  arc A1559 (-222.47, 0.63) -> (-222.3213, 0.7604) centre (-222.47, 0.78) ccw
  line L216 (-222.47, 0.63) -> (-222.9893, 0.63)
  arc A1560 (-223.138, 0.7604) -> (-222.9893, 0.63) centre (-222.9893, 0.78) ccw
  arc A1561 (-223.138, 0.7604) -> (-223.2306, 1.0682) centre (-224.1294, 0.63) ccw
  arc A1562 (-223.2306, 1.0682) -> (-223.7296, 1.38) centre (-223.7294, 0.825) ccw
  arc A1563 (-223.7296, 1.38) -> (-224.2287, 1.0682) centre (-223.7298, 0.825) ccw
  arc A1564 (-224.2287, 1.0682) -> (-224.3213, 0.7604) centre (-223.3298, 0.63) ccw
  arc A1565 (-224.47, 0.63) -> (-224.3213, 0.7604) centre (-224.47, 0.78) ccw
  line L217 (-224.47, 0.63) -> (-224.9893, 0.63)
  arc A1566 (-225.138, 0.7604) -> (-224.9893, 0.63) centre (-224.9893, 0.78) ccw
  arc A1567 (-225.138, 0.7604) -> (-225.2306, 1.0682) centre (-226.1294, 0.63) ccw
  arc A1568 (-225.2306, 1.0682) -> (-225.7296, 1.38) centre (-225.7294, 0.825) ccw
  arc A1569 (-225.7296, 1.38) -> (-226.2287, 1.0682) centre (-225.7298, 0.825) ccw
  arc A1570 (-226.2287, 1.0682) -> (-226.3213, 0.7604) centre (-225.3298, 0.63) ccw
  arc A1571 (-226.47, 0.63) -> (-226.3213, 0.7604) centre (-226.47, 0.78) ccw
  line L218 (-226.47, 0.63) -> (-226.9893, 0.63)
  arc A1572 (-227.138, 0.7604) -> (-226.9893, 0.63) centre (-226.9893, 0.78) ccw
  arc A1573 (-227.138, 0.7604) -> (-227.2306, 1.0682) centre (-228.1294, 0.63) ccw
  arc A1574 (-227.2306, 1.0682) -> (-227.7296, 1.38) centre (-227.7294, 0.825) ccw
  arc A1575 (-227.7296, 1.38) -> (-228.2287, 1.0682) centre (-227.7298, 0.825) ccw
  arc A1576 (-228.2287, 1.0682) -> (-228.3213, 0.7604) centre (-227.3298, 0.63) ccw
  arc A1577 (-228.47, 0.63) -> (-228.3213, 0.7604) centre (-228.47, 0.78) ccw
  line L219 (-228.47, 0.63) -> (-228.9893, 0.63)
  arc A1578 (-229.138, 0.7604) -> (-228.9893, 0.63) centre (-228.9893, 0.78) ccw
  arc A1579 (-229.138, 0.7604) -> (-229.2306, 1.0682) centre (-230.1294, 0.63) ccw
  arc A1580 (-229.2306, 1.0682) -> (-229.7296, 1.38) centre (-229.7294, 0.825) ccw
  arc A1581 (-229.7296, 1.38) -> (-230.2287, 1.0682) centre (-229.7298, 0.825) ccw
  arc A1582 (-230.2287, 1.0682) -> (-230.3213, 0.7604) centre (-229.3298, 0.63) ccw
  arc A1583 (-230.47, 0.63) -> (-230.3213, 0.7604) centre (-230.47, 0.78) ccw
  line L220 (-230.47, 0.63) -> (-230.9893, 0.63)
  arc A1584 (-231.138, 0.7604) -> (-230.9893, 0.63) centre (-230.9893, 0.78) ccw
  arc A1585 (-231.138, 0.7604) -> (-231.2306, 1.0682) centre (-232.1294, 0.63) ccw
  arc A1586 (-231.2306, 1.0682) -> (-231.7296, 1.38) centre (-231.7294, 0.825) ccw
  arc A1587 (-231.7296, 1.38) -> (-232.2287, 1.0682) centre (-231.7298, 0.825) ccw
  arc A1588 (-232.2287, 1.0682) -> (-232.3213, 0.7604) centre (-231.3298, 0.63) ccw
  arc A1589 (-232.47, 0.63) -> (-232.3213, 0.7604) centre (-232.47, 0.78) ccw
  line L221 (-232.47, 0.63) -> (-232.9893, 0.63)
  arc A1590 (-233.138, 0.7604) -> (-232.9893, 0.63) centre (-232.9893, 0.78) ccw
  arc A1591 (-233.138, 0.7604) -> (-233.2306, 1.0682) centre (-234.1294, 0.63) ccw
  arc A1592 (-233.2306, 1.0682) -> (-233.7296, 1.38) centre (-233.7294, 0.825) ccw
  arc A1593 (-233.7296, 1.38) -> (-234.2287, 1.0682) centre (-233.7298, 0.825) ccw
  arc A1594 (-234.2287, 1.0682) -> (-234.3213, 0.7604) centre (-233.3298, 0.63) ccw
  arc A1595 (-234.47, 0.63) -> (-234.3213, 0.7604) centre (-234.47, 0.78) ccw
  line L222 (-234.47, 0.63) -> (-234.9893, 0.63)
  arc A1596 (-235.138, 0.7604) -> (-234.9893, 0.63) centre (-234.9893, 0.78) ccw
  arc A1597 (-235.138, 0.7604) -> (-235.2306, 1.0682) centre (-236.1294, 0.63) ccw
  arc A1598 (-235.2306, 1.0682) -> (-235.7296, 1.38) centre (-235.7294, 0.825) ccw
  arc A1599 (-235.7296, 1.38) -> (-236.2287, 1.0682) centre (-235.7298, 0.825) ccw
  arc A1600 (-236.2287, 1.0682) -> (-236.3213, 0.7604) centre (-235.3298, 0.63) ccw
  arc A1601 (-236.47, 0.63) -> (-236.3213, 0.7604) centre (-236.47, 0.78) ccw
  line L223 (-236.47, 0.63) -> (-236.9893, 0.63)
  arc A1602 (-237.138, 0.7604) -> (-236.9893, 0.63) centre (-236.9893, 0.78) ccw
  arc A1603 (-237.138, 0.7604) -> (-237.2306, 1.0682) centre (-238.1294, 0.63) ccw
  arc A1604 (-237.2306, 1.0682) -> (-237.7296, 1.38) centre (-237.7294, 0.825) ccw
  arc A1605 (-237.7296, 1.38) -> (-238.2287, 1.0682) centre (-237.7298, 0.825) ccw
  arc A1606 (-238.2287, 1.0682) -> (-238.3213, 0.7604) centre (-237.3298, 0.63) ccw
  arc A1607 (-238.47, 0.63) -> (-238.3213, 0.7604) centre (-238.47, 0.78) ccw
  line L224 (-238.47, 0.63) -> (-238.9893, 0.63)
  arc A1608 (-239.138, 0.7604) -> (-238.9893, 0.63) centre (-238.9893, 0.78) ccw
  arc A1609 (-239.138, 0.7604) -> (-239.2306, 1.0682) centre (-240.1294, 0.63) ccw
  arc A1610 (-239.2306, 1.0682) -> (-239.7296, 1.38) centre (-239.7294, 0.825) ccw
  arc A1611 (-239.7296, 1.38) -> (-240.2287, 1.0682) centre (-239.7298, 0.825) ccw
  arc A1612 (-240.2287, 1.0682) -> (-240.3213, 0.7604) centre (-239.3298, 0.63) ccw
  arc A1613 (-240.47, 0.63) -> (-240.3213, 0.7604) centre (-240.47, 0.78) ccw
  line L225 (-240.47, 0.63) -> (-240.9893, 0.63)
  arc A1614 (-241.138, 0.7604) -> (-240.9893, 0.63) centre (-240.9893, 0.78) ccw
  arc A1615 (-241.138, 0.7604) -> (-241.2306, 1.0682) centre (-242.1294, 0.63) ccw
  arc A1616 (-241.2306, 1.0682) -> (-241.7296, 1.38) centre (-241.7294, 0.825) ccw
  arc A1617 (-241.7296, 1.38) -> (-242.2287, 1.0682) centre (-241.7298, 0.825) ccw
  arc A1618 (-242.2287, 1.0682) -> (-242.3213, 0.7604) centre (-241.3298, 0.63) ccw
  arc A1619 (-242.47, 0.63) -> (-242.3213, 0.7604) centre (-242.47, 0.78) ccw
  line L226 (-242.47, 0.63) -> (-242.9893, 0.63)
  arc A1620 (-243.138, 0.7604) -> (-242.9893, 0.63) centre (-242.9893, 0.78) ccw
  arc A1621 (-243.138, 0.7604) -> (-243.2306, 1.0682) centre (-244.1294, 0.63) ccw
  arc A1622 (-243.2306, 1.0682) -> (-243.7296, 1.38) centre (-243.7294, 0.825) ccw
  arc A1623 (-243.7296, 1.38) -> (-244.2287, 1.0682) centre (-243.7298, 0.825) ccw
  arc A1624 (-244.2287, 1.0682) -> (-244.3213, 0.7604) centre (-243.3298, 0.63) ccw
  arc A1625 (-244.47, 0.63) -> (-244.3213, 0.7604) centre (-244.47, 0.78) ccw
  line L227 (-244.47, 0.63) -> (-244.9893, 0.63)
  arc A1626 (-245.138, 0.7604) -> (-244.9893, 0.63) centre (-244.9893, 0.78) ccw
  arc A1627 (-245.138, 0.7604) -> (-245.2306, 1.0682) centre (-246.1294, 0.63) ccw
  arc A1628 (-245.2306, 1.0682) -> (-245.7296, 1.38) centre (-245.7294, 0.825) ccw
  arc A1629 (-245.7296, 1.38) -> (-246.2287, 1.0682) centre (-245.7298, 0.825) ccw
  arc A1630 (-246.2287, 1.0682) -> (-246.3213, 0.7604) centre (-245.3298, 0.63) ccw
  arc A1631 (-246.47, 0.63) -> (-246.3213, 0.7604) centre (-246.47, 0.78) ccw
  line L228 (-246.47, 0.63) -> (-246.9893, 0.63)
  arc A1632 (-247.138, 0.7604) -> (-246.9893, 0.63) centre (-246.9893, 0.78) ccw
  arc A1633 (-247.138, 0.7604) -> (-247.2306, 1.0682) centre (-248.1294, 0.63) ccw
  arc A1634 (-247.2306, 1.0682) -> (-247.7296, 1.38) centre (-247.7294, 0.825) ccw
  arc A1635 (-247.7296, 1.38) -> (-248.2287, 1.0682) centre (-247.7298, 0.825) ccw
  arc A1636 (-248.2287, 1.0682) -> (-248.3213, 0.7604) centre (-247.3298, 0.63) ccw
  arc A1637 (-248.47, 0.63) -> (-248.3213, 0.7604) centre (-248.47, 0.78) ccw
  line L229 (-248.47, 0.63) -> (-248.9893, 0.63)
  arc A1638 (-249.138, 0.7604) -> (-248.9893, 0.63) centre (-248.9893, 0.78) ccw
  arc A1639 (-249.138, 0.7604) -> (-249.2306, 1.0682) centre (-250.1294, 0.63) ccw
  arc A1640 (-249.2306, 1.0682) -> (-249.7296, 1.38) centre (-249.7294, 0.825) ccw
  arc A1641 (-249.7296, 1.38) -> (-250.2287, 1.0682) centre (-249.7298, 0.825) ccw
  arc A1642 (-250.2287, 1.0682) -> (-250.3213, 0.7604) centre (-249.3298, 0.63) ccw
  arc A1643 (-250.47, 0.63) -> (-250.3213, 0.7604) centre (-250.47, 0.78) ccw
  line L230 (-250.47, 0.63) -> (-250.9893, 0.63)
  arc A1644 (-251.138, 0.7604) -> (-250.9893, 0.63) centre (-250.9893, 0.78) ccw
  arc A1645 (-251.138, 0.7604) -> (-251.2306, 1.0682) centre (-252.1294, 0.63) ccw
  arc A1646 (-251.2306, 1.0682) -> (-251.7296, 1.38) centre (-251.7294, 0.825) ccw
  arc A1647 (-251.7296, 1.38) -> (-252.2287, 1.0682) centre (-251.7298, 0.825) ccw
  arc A1648 (-252.2287, 1.0682) -> (-252.3213, 0.7604) centre (-251.3298, 0.63) ccw
  arc A1649 (-252.47, 0.63) -> (-252.3213, 0.7604) centre (-252.47, 0.78) ccw
  line L231 (-252.47, 0.63) -> (-252.9893, 0.63)
  arc A1650 (-253.138, 0.7604) -> (-252.9893, 0.63) centre (-252.9893, 0.78) ccw
  arc A1651 (-253.138, 0.7604) -> (-253.2306, 1.0682) centre (-254.1294, 0.63) ccw
  arc A1652 (-253.2306, 1.0682) -> (-253.7296, 1.38) centre (-253.7294, 0.825) ccw
  arc A1653 (-253.7296, 1.38) -> (-254.2287, 1.0682) centre (-253.7298, 0.825) ccw
  arc A1654 (-254.2287, 1.0682) -> (-254.3213, 0.7604) centre (-253.3298, 0.63) ccw
  arc A1655 (-254.47, 0.63) -> (-254.3213, 0.7604) centre (-254.47, 0.78) ccw
  line L232 (-254.47, 0.63) -> (-254.9893, 0.63)
  arc A1656 (-255.138, 0.7604) -> (-254.9893, 0.63) centre (-254.9893, 0.78) ccw
  arc A1657 (-255.138, 0.7604) -> (-255.2306, 1.0682) centre (-256.1294, 0.63) ccw
  arc A1658 (-255.2306, 1.0682) -> (-255.7296, 1.38) centre (-255.7294, 0.825) ccw
  arc A1659 (-255.7296, 1.38) -> (-256.2287, 1.0682) centre (-255.7298, 0.825) ccw
  arc A1660 (-256.2287, 1.0682) -> (-256.3213, 0.7604) centre (-255.3298, 0.63) ccw
  arc A1661 (-256.47, 0.63) -> (-256.3213, 0.7604) centre (-256.47, 0.78) ccw
  line L233 (-256.47, 0.63) -> (-256.9893, 0.63)
  arc A1662 (-257.138, 0.7604) -> (-256.9893, 0.63) centre (-256.9893, 0.78) ccw
  arc A1663 (-257.138, 0.7604) -> (-257.2306, 1.0682) centre (-258.1294, 0.63) ccw
  arc A1664 (-257.2306, 1.0682) -> (-257.7296, 1.38) centre (-257.7294, 0.825) ccw
  arc A1665 (-257.7296, 1.38) -> (-258.2287, 1.0682) centre (-257.7298, 0.825) ccw
  arc A1666 (-258.2287, 1.0682) -> (-258.3213, 0.7604) centre (-257.3298, 0.63) ccw
  arc A1667 (-258.47, 0.63) -> (-258.3213, 0.7604) centre (-258.47, 0.78) ccw
  line L234 (-258.47, 0.63) -> (-258.9893, 0.63)
  arc A1668 (-259.138, 0.7604) -> (-258.9893, 0.63) centre (-258.9893, 0.78) ccw
  arc A1669 (-259.138, 0.7604) -> (-259.2306, 1.0682) centre (-260.1294, 0.63) ccw
  arc A1670 (-259.2306, 1.0682) -> (-259.7296, 1.38) centre (-259.7294, 0.825) ccw
  arc A1671 (-259.7296, 1.38) -> (-260.2287, 1.0682) centre (-259.7298, 0.825) ccw
  arc A1672 (-260.2287, 1.0682) -> (-260.3213, 0.7604) centre (-259.3298, 0.63) ccw
  arc A1673 (-260.47, 0.63) -> (-260.3213, 0.7604) centre (-260.47, 0.78) ccw
  line L235 (-260.47, 0.63) -> (-260.9893, 0.63)
  arc A1674 (-261.138, 0.7604) -> (-260.9893, 0.63) centre (-260.9893, 0.78) ccw
  arc A1675 (-261.138, 0.7604) -> (-261.2306, 1.0682) centre (-262.1294, 0.63) ccw
  arc A1676 (-261.2306, 1.0682) -> (-261.7296, 1.38) centre (-261.7294, 0.825) ccw
  arc A1677 (-261.7296, 1.38) -> (-262.2287, 1.0682) centre (-261.7298, 0.825) ccw
  arc A1678 (-262.2287, 1.0682) -> (-262.3213, 0.7604) centre (-261.3298, 0.63) ccw
  arc A1679 (-262.47, 0.63) -> (-262.3213, 0.7604) centre (-262.47, 0.78) ccw
  line L236 (-262.47, 0.63) -> (-262.9893, 0.63)
  arc A1680 (-263.138, 0.7604) -> (-262.9893, 0.63) centre (-262.9893, 0.78) ccw
  arc A1681 (-263.138, 0.7604) -> (-263.2306, 1.0682) centre (-264.1294, 0.63) ccw
  arc A1682 (-263.2306, 1.0682) -> (-263.7296, 1.38) centre (-263.7294, 0.825) ccw
  arc A1683 (-263.7296, 1.38) -> (-264.2287, 1.0682) centre (-263.7298, 0.825) ccw
  arc A1684 (-264.2287, 1.0682) -> (-264.3213, 0.7604) centre (-263.3298, 0.63) ccw
  arc A1685 (-264.47, 0.63) -> (-264.3213, 0.7604) centre (-264.47, 0.78) ccw
  line L237 (-264.47, 0.63) -> (-264.9893, 0.63)
  arc A1686 (-265.138, 0.7604) -> (-264.9893, 0.63) centre (-264.9893, 0.78) ccw
  arc A1687 (-265.138, 0.7604) -> (-265.2306, 1.0682) centre (-266.1294, 0.63) ccw
  arc A1688 (-265.2306, 1.0682) -> (-265.7296, 1.38) centre (-265.7294, 0.825) ccw
  arc A1689 (-265.7296, 1.38) -> (-266.2287, 1.0682) centre (-265.7298, 0.825) ccw
  arc A1690 (-266.2287, 1.0682) -> (-266.3213, 0.7604) centre (-265.3298, 0.63) ccw
  arc A1691 (-266.47, 0.63) -> (-266.3213, 0.7604) centre (-266.47, 0.78) ccw
  line L238 (-266.47, 0.63) -> (-266.9893, 0.63)
  arc A1692 (-267.138, 0.7604) -> (-266.9893, 0.63) centre (-266.9893, 0.78) ccw
  arc A1693 (-267.138, 0.7604) -> (-267.2306, 1.0682) centre (-268.1294, 0.63) ccw
  arc A1694 (-267.2306, 1.0682) -> (-267.7296, 1.38) centre (-267.7294, 0.825) ccw
  arc A1695 (-267.7296, 1.38) -> (-268.2287, 1.0682) centre (-267.7298, 0.825) ccw
  arc A1696 (-268.2287, 1.0682) -> (-268.3213, 0.7604) centre (-267.3298, 0.63) ccw
  arc A1697 (-268.47, 0.63) -> (-268.3213, 0.7604) centre (-268.47, 0.78) ccw
  line L239 (-268.47, 0.63) -> (-268.9893, 0.63)
  arc A1698 (-269.138, 0.7604) -> (-268.9893, 0.63) centre (-268.9893, 0.78) ccw
  arc A1699 (-269.138, 0.7604) -> (-269.2306, 1.0682) centre (-270.1294, 0.63) ccw
  arc A1700 (-269.2306, 1.0682) -> (-269.7296, 1.38) centre (-269.7294, 0.825) ccw
  arc A1701 (-269.7296, 1.38) -> (-270.2287, 1.0682) centre (-269.7298, 0.825) ccw
  arc A1702 (-270.2287, 1.0682) -> (-270.3213, 0.7604) centre (-269.3298, 0.63) ccw
  arc A1703 (-270.47, 0.63) -> (-270.3213, 0.7604) centre (-270.47, 0.78) ccw
  line L240 (-270.47, 0.63) -> (-270.9893, 0.63)
  arc A1704 (-271.138, 0.7604) -> (-270.9893, 0.63) centre (-270.9893, 0.78) ccw
  arc A1705 (-271.138, 0.7604) -> (-271.2306, 1.0682) centre (-272.1294, 0.63) ccw
  arc A1706 (-271.2306, 1.0682) -> (-271.7296, 1.38) centre (-271.7294, 0.825) ccw
  arc A1707 (-271.7296, 1.38) -> (-272.2287, 1.0682) centre (-271.7298, 0.825) ccw
  arc A1708 (-272.2287, 1.0682) -> (-272.3213, 0.7604) centre (-271.3298, 0.63) ccw
  arc A1709 (-272.47, 0.63) -> (-272.3213, 0.7604) centre (-272.47, 0.78) ccw